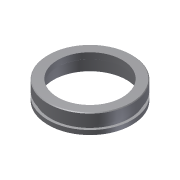
# Autodesk Inventor part: 鑄鐵SLEEVE
Saved by Autodesk Inventor 2012 SP2 (Build 160219200, 219)
## iProperties
Created: 2013-08-19
Part Number: 鑄鐵SLEEVE
Material: Default
Document SubType Name: Modeling
Designer: ERIC
Density: 1 g/cm^3
Author: ERIC
Autodesk Inventor part; units mm, degrees
ref_plane "YZ Plane" through (0, 0, 0) normal (1, 0, 0) x (0, 1, 0)
ref_plane "XZ Plane" through (0, 0, 0) normal (0, 1, 0) x (-1, 0, 0)
sketch "草圖1" plane through (0, 0, 0) normal (0, 0, 1) x (1, 0, 0)
  circle A0 centre (0, 0) radius 26
  dimension "d0" = 52
  constraints: 1 centre point, 1 coincident
  measures "d0" diameter of A0
extrude "擠出1" add sketch "草圖1" along normal blind 12.2
sketch "草圖2" plane through (0, 0, 12.2) normal (0, 0, 1) x (1, 0, 0)
  circle A0 centre (0, 0) radius 26 projected
  circle A1 centre (0, 0) radius 20
  dimension "d3" = 40
  constraints: 1 centre point, 1 coincident
  measures "d3" diameter of A1
extrude "擠出2" cut sketch "草圖2" against normal through all contours A1
sketch "草圖3" plane through (0, 0, 0) normal (0, 0, -1) x (-1, 0, 0)
  circle A0 centre (0, 0) radius 20 projected
  circle A1 centre (0, 0) radius 26 projected
  circle A2 centre (0, 0) radius 22.45
  dimension "d6" = 44.9
  constraints: 1 centre point, 1 coincident
  measures "d6" diameter of A2
extrude "擠出3" cut sketch "草圖3" against normal blind 8.2 contours A2
ref_plane "工作平面1" through (0, 0, 5.8) normal (0, 0, 1) x (1, 0, 0)
sketch "草圖4" plane through (0, 0, 5.8) normal (0, 0, 1) x (1, 0, 0)
  circle A0 centre (0, 0) radius 24.4
  circle A1 centre (0, 0) radius 26 projected
  dimension "d10" = 48.8
  constraints: 1 centre point, 1 coincident
  measures "d10" diameter of A0
extrude "擠出4" cut sketch "草圖4" against normal blind 2.8
chamfer "倒角1" distance 0.4 angle 45 3 edges at (-26, 0, 12.2) (-26, 0, 0) (22.45, 0, 0)
chamfer "倒角2" distance 0.3 angle 45 1 edges at (-20, 0, 8.2)
